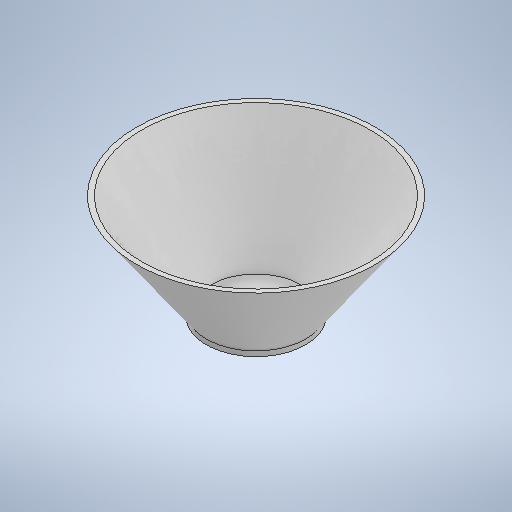
# Autodesk Inventor part: Lejek
Saved by Autodesk Inventor 2025 (Build 290162000, 162)
## iProperties
Created: 2024-12-31
Part Number: Lejek
Material: Ogólny
Document SubType Name: Modeling
Designer: Laptop
Density: 1 g/cm^3
Appearance: Domyślna
Author: Laptop
Autodesk Inventor part; units mm, degrees
ref_plane "YZ Plane" through (0, 0, 0) normal (1, 0, 0) x (0, 1, 0)
ref_plane "XZ Plane" through (0, 0, 0) normal (0, 1, 0) x (-1, 0, 0)
ref_plane "XY Plane" through (0, 0, 0) normal (0, 0, 1) x (1, 0, 0)
sketch "Szkic6" plane through (0, 0, 0) normal (0, 1, 0) x (-1, 0, 0)
  circle A0 centre (0, 0) radius 50
  dimension "d28" = 100
  constraints: 1 centre point, 1 coincident
  measures "d28" diameter of A0
extrude "Wyciągnięcie proste5" add sketch "Szkic6" along normal blind 100 draft 35
sketch "Szkic7" plane through (0, 0, 0) normal (0, -1, 0) x (1, 0, 0)
  circle A0 centre (0, 0) radius 45
  dimension "d31" = 90
  constraints: 1 centre point, 1 coincident
  measures "d31" diameter of A0
extrude "Wyciągnięcie proste6" cut sketch "Szkic7" against normal blind 100 draft 35
sketch "Szkic8" plane through (0, 0, 0) normal (0, -1, 0) x (1, 0, 0)
  circle A0 centre (0, 0) radius 50
  constraints: 1 centre point, 1 coincident
extrude "Wyciągnięcie proste7" add sketch "Szkic8" along normal blind 5
sketch "Szkic9" plane through (0, -5, 0) normal (0, -1, 0) x (1, 0, 0)
  circle A0 centre (0, 35) radius 2
  point P0 (0, 0)
  dimension "d36" = 4
  constraints: 1 centre point
  measures "d36" diameter of A0
extrude "Wyciągnięcie proste8" cut sketch "Szkic9" against normal blind 5
sketch "Szkic10" plane through (0, 0, 0) normal (0, 1, 0) x (1, 0, 0)
  circle A0 centre (0, 0) radius 5
  dimension "d39" = 10
  constraints: 1 centre point, 1 coincident
  measures "d39" diameter of A0
extrude "Wyciągnięcie proste9" cut sketch "Szkic10" against normal blind 5
